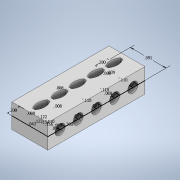
# Autodesk Inventor part: collimation_test
Saved by Autodesk Inventor 2022 (Build 260153000, 153)
## iProperties
Created: 2023-10-17
Part Number: collimation_test
Material: Generic
Document SubType Name: Modeling
Designer: William
Density: 1 g/cm^3
Appearance: Default
Author: William
Autodesk Inventor part; units mm, degrees
ref_plane "YZ Plane" through (0, 0, 0) normal (1, 0, 0) x (0, 1, 0)
ref_plane "XZ Plane" through (0, 0, 0) normal (0, 1, 0) x (-1, 0, 0)
ref_plane "XY Plane" through (0, 0, 0) normal (0, 0, 1) x (1, 0, 0)
sketch "Sketch1" plane through (0, 0, 0) normal (0, 1, 0) x (-1, 0, 0)
  line L0 (0, 0) -> (15, 0)
  line L1 (15, 0) -> (15, -40.64)
  line L2 (15, -40.64) -> (0, -40.64)
  line L3 (0, -40.64) -> (0, 0)
  line L4 (0, -5.08) -> (15, -5.08)
  line L5 (7.25, -1.98) -> (8.35, -1.98)
  line L6 (7.25, -8.18) -> (8.35, -8.18)
  arc A0 (8.35, -8.18) -> (8.35, -1.98) centre (4.045, -5.08) ccw
  arc A1 (7.25, -1.98) -> (7.25, -8.18) centre (11.555, -5.08) ccw
  line L7 (6.25, -5.08) -> (6.25, -4.52) construction
  line L8 (6.529761, -3.38) -> (9.070239, -3.38)
  line L9 (6.529761, -6.78) -> (9.070239, -6.78)
  line L10 (0, -12.7) -> (15, -12.7)
  arc A2 (8.35, -15.8) -> (8.35, -9.6) centre (4.045, -12.7) ccw
  line L11 (6.529761, -11) -> (9.070239, -11)
  line L12 (7.25, -9.6) -> (8.35, -9.6)
  line L13 (6.529761, -14.4) -> (9.070239, -14.4)
  line L14 (7.25, -15.8) -> (8.35, -15.8)
  arc A3 (7.25, -9.6) -> (7.25, -15.8) centre (11.555, -12.7) ccw
  line L15 (0, -20.32) -> (15, -20.32)
  arc A4 (8.35, -23.42) -> (8.35, -17.22) centre (4.045, -20.32) ccw
  line L16 (6.529761, -18.62) -> (9.070239, -18.62)
  line L17 (7.25, -17.22) -> (8.35, -17.22)
  line L18 (6.529761, -22.02) -> (9.070239, -22.02)
  line L19 (7.25, -23.42) -> (8.35, -23.42)
  arc A5 (7.25, -17.22) -> (7.25, -23.42) centre (11.555, -20.32) ccw
  line L20 (0, -27.94) -> (15, -27.94)
  arc A6 (8.35, -31.04) -> (8.35, -24.84) centre (4.045, -27.94) ccw
  line L21 (6.529761, -26.24) -> (9.070239, -26.24)
  line L22 (7.25, -24.84) -> (8.35, -24.84)
  line L23 (6.529761, -29.64) -> (9.070239, -29.64)
  line L24 (7.25, -31.04) -> (8.35, -31.04)
  arc A7 (7.25, -24.84) -> (7.25, -31.04) centre (11.555, -27.94) ccw
  line L25 (0, -35.56) -> (15, -35.56)
  arc A8 (8.35, -38.66) -> (8.35, -32.46) centre (4.045, -35.56) ccw
  line L26 (6.529761, -33.86) -> (9.070239, -33.86)
  line L27 (7.25, -32.46) -> (8.35, -32.46)
  line L28 (6.529761, -37.26) -> (9.070239, -37.26)
  line L29 (7.25, -38.66) -> (8.35, -38.66)
  arc A9 (7.25, -32.46) -> (7.25, -38.66) centre (11.555, -35.56) ccw
  line L30 (0, -7.18) -> (3.453771, -7.18)
  line L31 (3.453771, -7.18) -> (3.453771, -5.28)
  line L32 (3.453771, -5.28) -> (6.253771, -5.28)
  line L33 (15, -5.28) -> (9.346229, -5.28)
  line L34 (0, -14.8) -> (6.683345, -14.8)
  line L35 (9.346229, -12.9) -> (15, -12.9)
  line L36 (0, -22.42) -> (3.453771, -22.42)
  line L37 (3.453771, -22.42) -> (3.453771, -20.52)
  line L38 (3.453771, -20.52) -> (6.253771, -20.52)
  line L39 (15, -20.52) -> (9.070239, -22.02)
  line L40 (0, -30.04) -> (3.453771, -30.04)
  line L41 (3.453771, -30.04) -> (3.453771, -28.14)
  line L42 (3.453771, -28.14) -> (6.253771, -28.14)
  line L43 (15, -30.04) -> (8.916655, -30.04)
  line L44 (0, -37.66) -> (3.453771, -37.66)
  line L45 (3.453771, -37.66) -> (3.453771, -35.76)
  line L46 (3.453771, -35.76) -> (6.253771, -35.76)
  line L47 (9.346229, -35.76) -> (10.346229, -35.76)
  line L48 (10.346229, -35.76) -> (15, -38.66)
  point P0 (2.3, -5.08)
  point P1 (2.3, -12.7)
  point P2 (6.25, -12.7)
  point P3 (2.3, -20.32)
  point P4 (6.25, -20.32)
  point P5 (2.3, -27.94)
  point P6 (6.25, -27.94)
  point P7 (2.3, -35.56)
  point P8 (6.25, -35.56)
  dimension "d0" = 15
  dimension "d4" = 5.08
  dimension "d5" = 2.3
  dimension "d6" = 1.1
  dimension "d7" = 3.1
  dimension "d8" = 3.1
  dimension "d9" = 3.95
  dimension "d10" = 3.4
  dimension "d13" = 7.62
  dimension "d18" = 5.08
  dimension "d19" = 2.1
  dimension "d20" = 2.8
  dimension "d21" = 0.2
  dimension "d22" = 2.1
  dimension "d23" = 0.2
  dimension "d24" = 0.2
  dimension "d25" = 2.1
  dimension "d26" = 2.8
  dimension "d27" = 2.1
  dimension "d28" = 2.8
  dimension "d29" = 0.2
  dimension "d38" = 1
  dimension "d39" = 0.2
  dimension "d40" = 2.1
  dimension "d41" = 2.8
  constraints: 98 end point, 54 point on circle, 31 point on line, 11 horizontal, 10 centre point, 10 perpendicular, 5 parallel, 2 horizontal alignment, 2 vertical, 1 collinear, 1 equal radius, 1 tangent, 84 other
  measures "d0" distance of L1.end L2.end
  measures "d4" distance between parallel lines of L0 L4
  measures "d5" distance from line of L3 point (2.3, -5.08)
  measures "d6" distance of L5.start L5.end
  measures "d7" distance between parallel lines of L4 L5
  measures "d9" distance from line of point (2.3, -5.08) L7
  measures "d10" distance between parallel lines of L8 L9
  measures "d13" distance of L4.start L10.start
  measures "d18" distance between parallel lines of L2 L25
  measures "d19" distance between parallel lines of L30 L4
  measures "d20" distance of L31.end L32.end
  measures "d21" distance between parallel lines of L4 L33
  measures "d22" distance between parallel lines of L10 L34
  measures "d23" distance between parallel lines of L10 L35
  measures "d24" distance from line of L15 L39.start
  measures "d25" distance between parallel lines of L15 L36
  measures "d26" distance of L37.end L38.end
  measures "d27" distance between parallel lines of L20 L40
  measures "d28" distance of L41.end L42.end
  measures "d29" distance between parallel lines of L20 L42
  measures "d38" distance of L47.start L47.end
  measures "d39" distance between parallel lines of L25 L47
  measures "d40" distance between parallel lines of L25 L44
  measures "d41" distance of L45.end L46.end
extrude "Extrusion1" add sketch "Sketch1" along normal mid plane 10
extrude "Extrusion2" cut sketch "Sketch1" along normal mid plane 25.4 contours A1 L8 A0 L4 | L4 A0 L9 A1 | A3 L11 A2 L10 | L10 A2 L13 A3 | A5 L16 A4 L15 | L15 A4 L18 A5 | A7 L21 A6 L20 | L20 A6 L23 A7 | A9 L26 A8 L25 | L25 A8 L28 A9
extrude "Extrusion3" cut sketch "Sketch1" along normal blind 25.4 contours A1 L8 A0 L4 | L4 A0 L9 A1 | A1 L5 A0 L8 | A3 L11 A2 L10 | L10 A2 L13 A3 | L9 A0 L6 A1 | A3 L13 A2 L14 | A3 L12 A2 L11 | A5 L16 A4 L15 | L15 A4 L18 A5 | A5 L17 A4 L16 | A4 L19 A5 L18 | A7 L21 A6 L20 | L20 A6 L23 A7 | A7 L22 A6 L21 | A6 L24 A7 L23 | A9 L26 A8 L25 | L25 A8 L28 A9 | A9 L27 A8 L26 | L28 A8 L29 A9
revolve "Revolution1" cut sketch "Sketch1" angle 360 about axis through (0, 0, -5.08) along (-1, 0, 0) contours L4 A1 L32 L31 L30 L3 | L1 L33 A0 L4 | L4 A0 L9 A1 | L9 A0 L6 A1
revolve "Revolution2" cut sketch "Sketch1" angle 360 about axis through (0, 0, -12.7) along (-1, 0, 0) contours L10 A3 L34 L3 | L1 L35 A2 L10 | L10 A2 L13 A3 | A3 L13 A2 L14
revolve "Revolution3" cut sketch "Sketch1" angle 360 about axis through (0, 0, -20.32) along (-1, 0, 0) contours L15 A5 L38 L37 L36 L3 | L1 L39 A4 L15 | L15 A4 L18 A5 | A4 L19 A5 L18
revolve "Revolution4" cut sketch "Sketch1" angle 360 about axis through (0, 0, -27.94) along (-1, 0, 0) contours L20 A7 L42 L41 L40 L3 | L1 L43 A6 L20 | L20 A6 L23 A7 | A6 L24 A7 L23
revolve "Revolution5" cut sketch "Sketch1" angle 360 about axis through (0, 0, -35.56) along (-1, 0, 0) contours L25 A9 L46 L45 L44 L3 | L1 L48 L47 A8 L25 | L25 A8 L28 A9 | L28 A8 L29 A9
body "Solid1"
